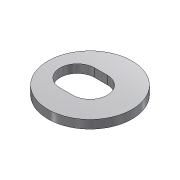
# Autodesk Inventor part: BC-10020
Saved by Autodesk Inventor 2016 (Build 200138000, 138)
## iProperties
Created: 2015-11-27
Part Number: BC-10020
Project: DIPOLO BC-3T- SIRIUS
Cost Center: 1504002005
Material: Aço Inox AISI 304
Document SubType Name: Modeling
Designer: reinaldo.basilio
Mass: 5.66287 g
Surface Area: 7.56156 cm^2
Volume: 0.707859 cm^3
Density: 8 g/cm^3
Appearance: Chrome - Satin
Description: Arruela.
RuleStatus: InUse
AfterMaterialChange0: file://_iMaterial
AfterAnyiPropertyChange0: file://_iMaterial
AfterDocNew0: file://_Naming_par
AfterDocNew1: file://_NameStart
AfterDocNew2: file://_NameStart1
AfterDocNew3: file://_Materiais
DocNumber: XXXXX-XXX-XXXX-00-001.ipt
Folder: .
Title: DIPOLO BC-3T- SIRIUS
Author: reinaldo.basilio
Subject: BC-10020
Autodesk Inventor part; units mm, degrees
ref_plane "YZ Plane" through (0, 0, 0) normal (1, 0, 0) x (0, 1, 0)
ref_plane "XZ Plane" through (0, 0, 0) normal (0, 1, 0) x (-1, 0, 0)
ref_plane "XY Plane" through (0, 0, 0) normal (0, 0, 1) x (1, 0, 0)
sketch "Sketch5" plane through (0, 0, 0) normal (0, 0, 1) x (1, 0, 0)
  circle A0 centre (0, 0) radius 10
  line L0 (0, 0) -> (0, -3) construction
  line L1 (-4.125, 0) -> (-4.125, -3)
  line L2 (4.125, -3) -> (4.125, 0)
  arc A1 (4.125, 0) -> (-4.125, 0) centre (0, 0) ccw
  arc A2 (-4.125, -3) -> (4.125, -3) centre (0, -3) ccw
  point P0 (0, -1.5)
  dimension "d8" = 20
  dimension "d9" = 8.25
  dimension "d10" = 3
  constraints: 8 end point, 4 point on circle, 4 tangent, 3 centre point, 1 coincident, 1 midpoint, 1 parallel, 1 vertical
  measures "d8" diameter of A0
  measures "d9" distance between parallel lines of L2 L1
  measures "d10" distance of L0.start L0.end
extrude "Extrusion5" add sketch "Sketch5" along normal blind 2
body "Solid5"
